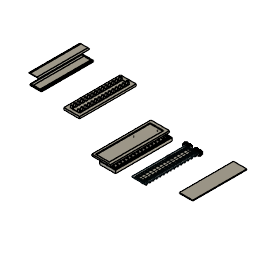
Prototype_caterpillar_body_mold_asser v11 (Autodesk Fusion 360 design; units mm, degrees)
Autodesk Fusion 360 part; units mm, degrees
note: some values were not read from the file. Chosen so that the rebuilt part matches the saved one: which bodies a step acts on; which face or edge a step refers to. Set by a fixed rule: which sketch regions a step uses.
(part 1 of 3)
sketch "Sketch1" plane through (0, 0, 0) normal (1, 0, 0) x (0, 1, 0)
  line L0 (0, 0) -> (0, 15)
  line L1 (0, 0) -> (5, 0)
  line L2 (5, 0) -> (13.6603, 15)
  line L3 (13.6603, 15) -> (16.3397, 15)
  line L4 (16.3397, 15) -> (25, 0)
  line L5 (25, 0) -> (30, 0)
  line L6 (30, 0) -> (38.6605, 15.0004)
  line L7 (0, 15) -> (38.6605, 15.0004)
  line L8 (12.7943, 13.5001) -> (17.2057, 13.5002)
  line L9 (12.7943, 13.5001) -> (12.7943, 15.0001)
  dimension "d1" = 15
  dimension "d4" = 5
  dimension "d5" = 120
  dimension "d9" = 15
  dimension "d11" = 120
  dimension "d12" = 20
  dimension "d13" = 5
  dimension "d14" = 2.6795
  dimension "d15" = 120
  dimension "d16" = 17.321
  dimension "d17" = 1.5
  constraint coincident L0.start L1.start
  constraint vertical L0
  constraint perpendicular L0 L1
  constraint perpendicular L0 L3
  constraint horizontal L5
  constraint coincident L2 L8.start
  constraint coincident L4 L8.end
  constraint parallel L7 L8
  constraint coincident L7 L9.end
  constraint perpendicular L7 L9
  measures "d1" distance of L0.start L0.end
  measures "d4" distance of L0.start L1.end
  measures "d5" angle of L1 L2
  measures "d9" distance of L1 L3
  measures "d11" angle of L4 L5
  measures "d12" distance of L1.end L4.end
  measures "d13" distance of L4.end L5.end
  measures "d14" distance of L2.end L3.end
  measures "d15" angle of L5 L6
  measures "d16" distance of L5.end L6.end
  measures "d17" distance of L7 L8
extrude "Extrude1" add sketch "Sketch1" along normal blind 60 contours L2 L7 L9 | L2 L3 L4 L7 L8 | L4 L5 L6 L7 makes body 1
sketch "Sketch2" plane through (0, 0, 0) normal (0, -1, 0) x (1, 0, 0)
  line L0 (0, 15) -> (0, 0)
  line L1 (0, 0) -> (60, 0)
  line L2 (60, 0) -> (60, 15)
  line L3 (60, 15) -> (0, 15)
  line L4 (0, 0) -> (15, 0)
  line L5 (60, 0) -> (45, 0)
  line L6 (15, 0) -> (30, 13.5)
  line L7 (45, 0) -> (30, 13.5)
  line L8 (15, 0) -> (45, 0)
  dimension "d23" = 15
  dimension "d24" = 15
  dimension "d28" = 138.013
  dimension "d29" = 138.013
  constraint coincident L0.end L1.start
  constraint coincident L1 L4.end
  constraint perpendicular L2 L4
  constraint coincident L1.end L2.start
  constraint coincident L1 L5.end
  constraint perpendicular L2 L5
  measures "d23" distance of L0.end L4.end
  measures "d24" distance of L1.end L5.end
  measures "d28" angle of L4 L6
  measures "d29" angle of L5 L7
extrude "Extrude2" cut sketch "Sketch2" along normal through all and the other way through all contours L1 L6 L7 L8 bodies 1
sketch "Sketch5" plane through (60, 0, 0) normal (1, 0, 0) x (0, 1, 0)
  line L0 (17.2057, 13.5002) -> (25, 0)
  line L1 (25, 0) -> (30, 0)
  line L2 (30, 0) -> (38.6605, 15.0004)
  line L3 (38.6605, 15.0004) -> (12.7943, 15.0001)
  line L4 (12.7943, 15.0001) -> (12.7943, 13.5001)
  line L5 (12.7943, 13.5001) -> (17.2057, 13.5002)
  line L6 (18.649, 15.0002) -> (24.7114, 4.4999)
  line L7 (24.7114, 4.4999) -> (30.2887, 4.5)
  line L8 (30.2887, 4.5) -> (36.3511, 15.0004)
  line L9 (18.649, 15.0002) -> (36.3511, 15.0004)
  dimension "d32" = 2
  dimension "d33" = 2
  dimension "d35" = 4.5
  constraint coincident L3 L6.start
  constraint parallel L3 L7
  constraint parallel L0 L6
  constraint parallel L2 L8
  constraint coincident L3 L8.end
  measures "d32" distance of L0 L6
  measures "d33" distance of L2 L8
  measures "d35" distance of L1.end L7
extrude "Extrude3" cut sketch "Sketch5" against normal blind 11 from surface at -4 contours L3 L6 L7 L8 L9 bodies 1
ref_plane "WorkPlane1" through (30, 25.7274, 7.5002) normal (1, 0, 0) x (0, 0, -1)
mirror "Mirror1" about plane through (30, 25.7274, 7.5002) normal (1, 0, 0) of "Extrude3"
pattern_linear "R-Pattern1" count 10 spacing 25 along (0, 1, 0) of bodies 1 makes body 2 at (35, 55.4504, 15.0003) makes body 3 at (35, 80.4504, 15.0003) makes body 4 at (35, 105.4504, 15.0003) makes body 5 at (35, 130.4504, 15.0003) makes body 6 at (35, 155.4504, 15.0003) makes body 7 at (35, 180.4504, 15.0003) makes body 8 at (35, 205.4504, 15.0003) makes body 9 at (35, 230.4504, 15.0003) makes body 10 at (35, 249.5497, 15.0003)
combine "Combine1" operation add target body 1 tool bodies 2 3 4 5 6 7 8 10 9
extrude "Extrude4" add sketch "Sketch1" along normal up to surface (60 mm away) contours L0 L1 L2 L7 L9 bodies 1
sketch "Sketch6" plane through (0, -0.0002, 15) normal (0, -0.000011, 1) x (1, 0, 0)
  line L0 (15, 18.6492) -> (4, 18.6492)
  line L1 (4, 18.6492) -> (4, 36.3512)
  line L2 (4, 36.3512) -> (15, 36.3512)
  line L3 (15, 36.3512) -> (15, 18.6492)
  line L4 (56, 18.6492) -> (45, 18.6492)
  line L5 (45, 18.6492) -> (45, 36.3512)
  line L6 (45, 36.3512) -> (56, 36.3512)
  line L7 (56, 36.3512) -> (56, 18.6492)
  line L8 (0, 38.6607) -> (0, 0.0002)
  line L9 (0, 0.0002) -> (60, 0.0002)
  line L10 (60, 0.0002) -> (60, 38.6607)
  line L11 (60, 38.6607) -> (0, 38.6607)
  line L12 (51.5, 36.3512) -> (49.5, 36.3512)
  line L13 (49.5, 36.3512) -> (49.5, 243.65)
  line L14 (49.5, 243.65) -> (51.5, 243.65)
  line L15 (51.5, 243.65) -> (51.5, 36.3512)
  line L16 (56, 243.65) -> (54.86, 243.65)
  line L17 (0, 263.5) -> (60, 263.5)
  line L18 (30, 263.5) -> (30, 202.2407)
  line L19 (8.5, 243.65) -> (8.5, 36.3512)
  line L20 (10.5, 36.3512) -> (10.5, 243.65)
  line L21 (8.5, 36.3512) -> (10.5, 36.3512)
  line L22 (10.5, 243.65) -> (8.5, 243.65)
  dimension "d48" = 2
  constraint vertical L13
  constraint horizontal L14
  constraint vertical L15
  constraint collinear L6 L12
  constraint horizontal L16
  constraint collinear L14 L16
  constraint midpoint L6 L12
  constraint horizontal L17
  constraint midpoint L17 L18.start
  constraint perpendicular L17 L18
  constraint symmetric L12.start L18 L19.end
  constraint symmetric L12.end L18 L20.start
  constraint symmetric L13.end L18 L20.end
  constraint symmetric L14.end L18 L19.start
  measures "d48" distance of L12.start L12.end
extrude "Extrude5" cut sketch "Sketch6" against normal blind 1 contours L2 L11 L19 L20 L21 | L11 L19 L20 L22 | L11 L13 L14 L15 | L6 L11 L12 L13 L15 bodies 1
extrude "Extrude6" add sketch "Sketch2" along normal blind 5 contours L0 L1 L2 L3 L4 L5 L6 L7 bodies 1
extrude "Extrude7" cut sketch "Sketch2" against normal blind 150 contours L1 L6 L7 L8 bodies 1
sketch "Sketch7" plane through (0, -0.0002, 15) normal (0, -0.000011, 1) x (1, 0, 0)
  line L0 (8.5, 36.3512) -> (8.5, 38.6607)
  line L1 (8.5, 38.6607) -> (0, 38.6607)
  line L2 (0, 38.6607) -> (0, 0.0002)
  line L3 (0, 0.0002) -> (60, 0.0002)
  line L4 (60, 0.0002) -> (60, 38.6607)
  line L5 (60, 38.6607) -> (51.5, 38.6607)
  line L6 (51.5, 38.6607) -> (51.5, 36.3512)
  line L7 (51.5, 36.3512) -> (56, 36.3512)
  line L8 (56, 36.3512) -> (56, 18.6492)
  line L9 (56, 18.6492) -> (45, 18.6492)
  line L10 (45, 18.6492) -> (45, 36.3512)
  line L11 (45, 36.3512) -> (49.5, 36.3512)
  line L12 (49.5, 36.3512) -> (49.5, 38.6607)
  line L13 (49.5, 38.6607) -> (10.5, 38.6607)
  line L14 (10.5, 38.6607) -> (10.5, 36.3512)
  line L15 (10.5, 36.3512) -> (15, 36.3512)
  line L16 (15, 36.3512) -> (15, 18.6492)
  line L17 (15, 18.6492) -> (4, 18.6492)
  line L18 (4, 18.6492) -> (4, 36.3512)
  line L19 (4, 36.3512) -> (8.5, 36.3512)
  line L20 (56, 18.6492) -> (45, 18.6492)
  line L21 (45, 18.6492) -> (45, 261.35)
  line L22 (45, 261.35) -> (56, 261.35)
  line L23 (56, 261.35) -> (56, 18.6492)
  line L24 (15, 18.6492) -> (4, 18.6492)
  line L25 (4, 18.6492) -> (4, 261.3513)
  line L26 (4, 261.3513) -> (15, 261.3513)
  line L27 (15, 261.3513) -> (15, 18.6492)
  line L28 (57, 262.35) -> (57, 17.6492)
  line L29 (57, 17.6492) -> (44, 17.6492)
  line L30 (44, 17.6492) -> (44, 262.35)
  line L31 (44, 262.35) -> (57, 262.35)
  line L32 (3, 262.3513) -> (16, 262.3513)
  line L33 (16, 262.3513) -> (16, 17.6492)
  line L34 (16, 17.6492) -> (3, 17.6492)
  line L35 (3, 17.6492) -> (3, 262.3513)
  dimension "d56" = -1
  dimension "d57" = -1
  constraint horizontal L20
  constraint vertical L21
  constraint horizontal L22
  constraint vertical L23
  constraint coincident L8.end L9.start
  constraint horizontal L24
  constraint vertical L25
  constraint horizontal L26
  constraint vertical L27
  constraint coincident L16.end L17.start
extrude "Extrude8" add sketch "Sketch7" along normal blind 2 contours L1 L13 L16 L17 L18 L24 L25 L27 L33 L34 L35 | L1 L13 L25 L26 L27 L32 L33 L35 | L5 L13 L21 L22 L23 L28 L30 L31 | L5 L8 L9 L10 L13 L20 L21 L23 L28 L29 L30 bodies 1
sketch "Sketch8" plane through (0, -0.0002, 14.9997) normal (0, -0.000011, 1) x (1, 0, 0)
  line L0 (8.5, 61.3512) -> (8.5, 63.6607)
  line L1 (8.5, 63.6607) -> (0, 63.6607)
  line L2 (0, 63.6607) -> (0, 38.6605)
  line L3 (0, 38.6605) -> (8.5, 38.6605)
  line L4 (8.5, 38.6605) -> (8.5, 43.6492)
  line L5 (8.5, 43.6492) -> (4, 43.6492)
  line L6 (4, 43.6492) -> (4, 61.3512)
  line L7 (4, 61.3512) -> (8.5, 61.3512)
  line L8 (8.5, 36.35) -> (4, 36.35)
  line L9 (4, 36.35) -> (4, 43.6492)
  line L10 (4, 43.6492) -> (8.5, 43.6492)
  line L11 (8.5, 43.6492) -> (8.5, 36.35)
  line L12 (4, 43.6492) -> (4, 36.35)
  line L13 (5, 42.6492) -> (7.5, 42.6492)
  line L14 (7.5, 42.6492) -> (7.5, 37.35)
  line L15 (7.5, 37.35) -> (5, 37.35)
  line L16 (5, 37.35) -> (5, 42.6492)
  line L17 (15, 19) -> (4, 19)
  line L18 (9.5, 19) -> (9.5, 28.6164)
  line L19 (11.5, 37.35) -> (14, 37.35)
  line L20 (14, 42.6492) -> (11.5, 42.6492)
  line L21 (14, 37.35) -> (14, 42.6492)
  line L22 (11.5, 42.6492) -> (11.5, 37.35)
  line L23 (60, 0) -> (0, 0)
  line L24 (30, 0) -> (30, 31)
  line L25 (0, 63.6605) -> (8.5, 63.6605)
  line L26 (8.5, 63.6605) -> (8.5, 68.6492)
  line L27 (11.5, 62.35) -> (14, 62.35)
  line L28 (8.5, 68.6492) -> (4, 68.6492)
  line L29 (5, 67.6492) -> (7.5, 67.6492)
  line L30 (7.5, 62.35) -> (5, 62.35)
  line L31 (5, 62.35) -> (5, 67.6492)
  line L32 (4, 68.6492) -> (8.5, 68.6492)
  line L33 (14, 67.6492) -> (11.5, 67.6492)
  line L34 (8.5, 61.35) -> (4, 61.35)
  line L35 (14, 62.35) -> (14, 67.6492)
  line L36 (8.5, 68.6492) -> (8.5, 61.35)
  line L37 (4, 68.6492) -> (4, 61.35)
  line L38 (11.5, 67.6492) -> (11.5, 62.35)
  line L39 (7.5, 67.6492) -> (7.5, 62.35)
  line L40 (4, 61.35) -> (4, 68.6492)
  line L41 (0, 88.6605) -> (8.5, 88.6605)
  line L42 (8.5, 88.6605) -> (8.5, 93.6492)
  line L43 (11.5, 87.35) -> (14, 87.35)
  line L44 (8.5, 93.6492) -> (4, 93.6492)
  line L45 (5, 92.6492) -> (7.5, 92.6492)
  line L46 (7.5, 87.35) -> (5, 87.35)
  line L47 (5, 87.35) -> (5, 92.6492)
  line L48 (4, 93.6492) -> (8.5, 93.6492)
  line L49 (14, 92.6492) -> (11.5, 92.6492)
  line L50 (8.5, 86.35) -> (4, 86.35)
  line L51 (14, 87.35) -> (14, 92.6492)
  line L52 (8.5, 93.6492) -> (8.5, 86.35)
  line L53 (4, 93.6492) -> (4, 86.35)
  line L54 (11.5, 92.6492) -> (11.5, 87.35)
  line L55 (7.5, 92.6492) -> (7.5, 87.35)
  line L56 (4, 86.35) -> (4, 93.6492)
  line L57 (0, 113.6605) -> (8.5, 113.6605)
  line L58 (8.5, 113.6605) -> (8.5, 118.6492)
  line L59 (11.5, 112.35) -> (14, 112.35)
  line L60 (8.5, 118.6492) -> (4, 118.6492)
  line L61 (5, 117.6492) -> (7.5, 117.6492)
  line L62 (7.5, 112.35) -> (5, 112.35)
  line L63 (5, 112.35) -> (5, 117.6492)
  line L64 (4, 118.6492) -> (8.5, 118.6492)
  line L65 (14, 117.6492) -> (11.5, 117.6492)
  line L66 (8.5, 111.35) -> (4, 111.35)
  line L67 (14, 112.35) -> (14, 117.6492)
  line L68 (8.5, 118.6492) -> (8.5, 111.35)
  line L69 (4, 118.6492) -> (4, 111.35)
  line L70 (11.5, 117.6492) -> (11.5, 112.35)
  line L71 (7.5, 117.6492) -> (7.5, 112.35)
  line L72 (4, 111.35) -> (4, 118.6492)
  line L73 (0, 138.6605) -> (8.5, 138.6605)
  line L74 (8.5, 138.6605) -> (8.5, 143.6492)
  line L75 (11.5, 137.35) -> (14, 137.35)
  line L76 (8.5, 143.6492) -> (4, 143.6492)
  line L77 (5, 142.6492) -> (7.5, 142.6492)
  line L78 (7.5, 137.35) -> (5, 137.35)
  line L79 (5, 137.35) -> (5, 142.6492)
  line L80 (4, 143.6492) -> (8.5, 143.6492)
  line L81 (14, 142.6492) -> (11.5, 142.6492)
  line L82 (8.5, 136.35) -> (4, 136.35)
  line L83 (14, 137.35) -> (14, 142.6492)
  line L84 (8.5, 143.6492) -> (8.5, 136.35)
  line L85 (4, 143.6492) -> (4, 136.35)
  line L86 (11.5, 142.6492) -> (11.5, 137.35)
  line L87 (7.5, 142.6492) -> (7.5, 137.35)
  line L88 (4, 136.35) -> (4, 143.6492)
  line L89 (0, 163.6605) -> (8.5, 163.6605)
  line L90 (8.5, 163.6605) -> (8.5, 168.6492)
  line L91 (11.5, 162.35) -> (14, 162.35)
  line L92 (8.5, 168.6492) -> (4, 168.6492)
  line L93 (5, 167.6492) -> (7.5, 167.6492)
  line L94 (7.5, 162.35) -> (5, 162.35)
  line L95 (5, 162.35) -> (5, 167.6492)
  line L96 (4, 168.6492) -> (8.5, 168.6492)
  line L97 (14, 167.6492) -> (11.5, 167.6492)
  line L98 (8.5, 161.35) -> (4, 161.35)
  line L99 (14, 162.35) -> (14, 167.6492)
  line L100 (8.5, 168.6492) -> (8.5, 161.35)
  line L101 (4, 168.6492) -> (4, 161.35)
  line L102 (11.5, 167.6492) -> (11.5, 162.35)
  line L103 (7.5, 167.6492) -> (7.5, 162.35)
  line L104 (4, 161.35) -> (4, 168.6492)
  line L105 (0, 188.6605) -> (8.5, 188.6605)
  line L106 (8.5, 188.6605) -> (8.5, 193.6492)
  line L107 (11.5, 187.35) -> (14, 187.35)
  line L108 (8.5, 193.6492) -> (4, 193.6492)
  line L109 (5, 192.6492) -> (7.5, 192.6492)
  line L110 (7.5, 187.35) -> (5, 187.35)
  line L111 (5, 187.35) -> (5, 192.6492)
  line L112 (4, 193.6492) -> (8.5, 193.6492)
  line L113 (14, 192.6492) -> (11.5, 192.6492)
  line L114 (8.5, 186.35) -> (4, 186.35)
  line L115 (14, 187.35) -> (14, 192.6492)
  line L116 (8.5, 193.6492) -> (8.5, 186.35)
  line L117 (4, 193.6492) -> (4, 186.35)
  line L118 (11.5, 192.6492) -> (11.5, 187.35)
  line L119 (7.5, 192.6492) -> (7.5, 187.35)
  line L120 (4, 186.35) -> (4, 193.6492)
  line L121 (0, 213.6605) -> (8.5, 213.6605)
  line L122 (8.5, 213.6605) -> (8.5, 218.6492)
  line L123 (11.5, 212.35) -> (14, 212.35)
  line L124 (8.5, 218.6492) -> (4, 218.6492)
  line L125 (5, 217.6492) -> (7.5, 217.6492)
  line L126 (7.5, 212.35) -> (5, 212.35)
  line L127 (5, 212.35) -> (5, 217.6492)
  line L128 (4, 218.6492) -> (8.5, 218.6492)
  line L129 (14, 217.6492) -> (11.5, 217.6492)
  line L130 (8.5, 211.35) -> (4, 211.35)
  line L131 (14, 212.35) -> (14, 217.6492)
  line L132 (8.5, 218.6492) -> (8.5, 211.35)
  line L133 (4, 218.6492) -> (4, 211.35)
  line L134 (11.5, 217.6492) -> (11.5, 212.35)
  line L135 (7.5, 217.6492) -> (7.5, 212.35)
  line L136 (4, 211.35) -> (4, 218.6492)
  line L137 (0, 238.6605) -> (8.5, 238.6605)
  line L138 (8.5, 238.6605) -> (8.5, 243.6492)
  line L139 (11.5, 237.35) -> (14, 237.35)
  line L140 (8.5, 243.6492) -> (4, 243.6492)
  line L141 (5, 242.6492) -> (7.5, 242.6492)
  line L142 (7.5, 237.35) -> (5, 237.35)
  line L143 (5, 237.35) -> (5, 242.6492)
  line L144 (4, 243.6492) -> (8.5, 243.6492)
  line L145 (14, 242.6492) -> (11.5, 242.6492)
  line L146 (8.5, 236.35) -> (4, 236.35)
  line L147 (14, 237.35) -> (14, 242.6492)
  line L148 (8.5, 243.6492) -> (8.5, 236.35)
  line L149 (4, 243.6492) -> (4, 236.35)
  line L150 (11.5, 242.6492) -> (11.5, 237.35)
  line L151 (7.5, 242.6492) -> (7.5, 237.35)
  line L152 (4, 236.35) -> (4, 243.6492)
  line L153 (45, 19) -> (56, 19)
  line L154 (48.5, 37.35) -> (46, 37.35)
  line L155 (56, 93.6492) -> (56, 86.35)
  line L156 (52.5, 187.35) -> (55, 187.35)
  line L157 (56, 118.6492) -> (56, 111.35)
  line L158 (46, 187.35) -> (46, 192.6492)
  line L159 (51.5, 136.35) -> (56, 136.35)
  line L160 (52.5, 37.35) -> (55, 37.35)
  line L161 (52.5, 167.6492) -> (52.5, 162.35)
  line L162 (56, 43.6492) -> (56, 36.35)
  line L163 (51.5, 118.6492) -> (51.5, 111.35)
  line L164 (55, 37.35) -> (55, 42.6492)
  line L165 (51.5, 61.3512) -> (51.5, 63.6607)
  line L166 (60, 113.6605) -> (51.5, 113.6605)
  line L167 (51.5, 88.6605) -> (51.5, 93.6492)
  line L168 (56, 61.3512) -> (51.5, 61.3512)
  line L169 (52.5, 42.6492) -> (52.5, 37.35)
  line L170 (48.5, 142.6492) -> (48.5, 137.35)
  line L171 (55, 237.35) -> (55, 242.6492)
  line L172 (51.5, 43.6492) -> (51.5, 36.35)
  line L173 (51.5, 63.6607) -> (60, 63.6607)
  line L174 (46, 42.6492) -> (48.5, 42.6492)
  line L175 (60, 163.6605) -> (51.5, 163.6605)
  line L176 (51.5, 86.35) -> (56, 86.35)
  line L177 (56, 143.6492) -> (56, 136.35)
  line L178 (50.5, 19) -> (50.5, 28.6164)
  line L179 (55, 167.6492) -> (52.5, 167.6492)
  line L180 (60, 38.6605) -> (51.5, 38.6605)
  line L181 (51.5, 188.6605) -> (51.5, 193.6492)
  line L182 (51.5, 36.35) -> (56, 36.35)
  line L183 (56, 168.6492) -> (56, 161.35)
  line L184 (48.5, 87.35) -> (46, 87.35)
  line L185 (46, 112.35) -> (46, 117.6492)
  line L186 (51.5, 138.6605) -> (51.5, 143.6492)
  line L187 (56, 36.35) -> (56, 43.6492)
  line L188 (55, 42.6492) -> (52.5, 42.6492)
  line L189 (46, 167.6492) -> (48.5, 167.6492)
  line L190 (51.5, 38.6605) -> (51.5, 43.6492)
  line L191 (51.5, 111.35) -> (56, 111.35)
  line L192 (56, 143.6492) -> (51.5, 143.6492)
  line L193 (48.5, 112.35) -> (46, 112.35)
  line L194 (46, 37.35) -> (46, 42.6492)
  line L195 (51.5, 43.6492) -> (56, 43.6492)
  line L196 (56, 43.6492) -> (51.5, 43.6492)
  line L197 (52.5, 112.35) -> (55, 112.35)
  line L198 (48.5, 137.35) -> (46, 137.35)
  line L199 (60, 188.6605) -> (51.5, 188.6605)
  line L200 (60, 138.6605) -> (51.5, 138.6605)
  line L201 (60, 63.6607) -> (60, 38.6605)
  line L202 (56, 43.6492) -> (56, 61.3512)
  line L203 (48.5, 42.6492) -> (48.5, 37.35)
  line L204 (56, 168.6492) -> (51.5, 168.6492)
  line L205 (55, 187.35) -> (55, 192.6492)
  line L206 (55, 192.6492) -> (52.5, 192.6492)
  line L207 (56, 86.35) -> (56, 93.6492)
  line L208 (52.5, 237.35) -> (55, 237.35)
  line L209 (46, 237.35) -> (46, 242.6492)
  line L210 (48.5, 162.35) -> (46, 162.35)
  line L211 (56, 193.6492) -> (51.5, 193.6492)
  line L212 (48.5, 242.6492) -> (48.5, 237.35)
  line L213 (52.5, 137.35) -> (55, 137.35)
  line L214 (55, 112.35) -> (55, 117.6492)
  line L215 (51.5, 193.6492) -> (56, 193.6492)
  line L216 (52.5, 142.6492) -> (52.5, 137.35)
  line L217 (51.5, 218.6492) -> (51.5, 211.35)
  line L218 (46, 192.6492) -> (48.5, 192.6492)
  line L219 (55, 142.6492) -> (52.5, 142.6492)
  line L220 (52.5, 117.6492) -> (52.5, 112.35)
  line L221 (56, 243.6492) -> (51.5, 243.6492)
  line L222 (48.5, 117.6492) -> (48.5, 112.35)
  line L223 (51.5, 163.6605) -> (51.5, 168.6492)
  line L224 (56, 243.6492) -> (56, 236.35)
  line L225 (48.5, 217.6492) -> (48.5, 212.35)
  line L226 (46, 242.6492) -> (48.5, 242.6492)
  line L227 (55, 87.35) -> (55, 92.6492)
  line L228 (46, 162.35) -> (46, 167.6492)
  line L229 (52.5, 212.35) -> (55, 212.35)
  line L230 (51.5, 68.6492) -> (56, 68.6492)
  line L231 (60, 63.6605) -> (51.5, 63.6605)
  line L232 (52.5, 242.6492) -> (52.5, 237.35)
  line L233 (46, 117.6492) -> (48.5, 117.6492)
  line L234 (52.5, 162.35) -> (55, 162.35)
  line L235 (55, 137.35) -> (55, 142.6492)
  line L236 (55, 117.6492) -> (52.5, 117.6492)
  line L237 (46, 212.35) -> (46, 217.6492)
  line L238 (51.5, 213.6605) -> (51.5, 218.6492)
  line L239 (51.5, 186.35) -> (56, 186.35)
  line L240 (52.5, 92.6492) -> (52.5, 87.35)
  line L241 (48.5, 192.6492) -> (48.5, 187.35)
  line L242 (46, 87.35) -> (46, 92.6492)
  line L243 (51.5, 238.6605) -> (51.5, 243.6492)
  line L244 (46, 142.6492) -> (48.5, 142.6492)
  line L245 (51.5, 143.6492) -> (56, 143.6492)
  line L246 (56, 186.35) -> (56, 193.6492)
  line L247 (56, 161.35) -> (56, 168.6492)
  line L248 (56, 193.6492) -> (56, 186.35)
  line L249 (56, 111.35) -> (56, 118.6492)
  line L250 (51.5, 168.6492) -> (56, 168.6492)
  line L251 (52.5, 192.6492) -> (52.5, 187.35)
  line L252 (55, 162.35) -> (55, 167.6492)
  line L253 (48.5, 187.35) -> (46, 187.35)
  line L254 (56, 118.6492) -> (51.5, 118.6492)
  line L255 (55, 212.35) -> (55, 217.6492)
  line L256 (56, 136.35) -> (56, 143.6492)
  line L257 (55, 217.6492) -> (52.5, 217.6492)
  line L258 (51.5, 193.6492) -> (51.5, 186.35)
  line L259 (56, 218.6492) -> (56, 211.35)
  line L260 (52.5, 67.6492) -> (52.5, 62.35)
  line L261 (51.5, 243.6492) -> (56, 243.6492)
  line L262 (51.5, 143.6492) -> (51.5, 136.35)
  line L263 (51.5, 236.35) -> (56, 236.35)
  line L264 (46, 67.6492) -> (48.5, 67.6492)
  line L265 (56, 68.6492) -> (56, 61.35)
  line L266 (48.5, 167.6492) -> (48.5, 162.35)
  line L267 (55, 92.6492) -> (52.5, 92.6492)
  line L268 (51.5, 168.6492) -> (51.5, 161.35)
  line L269 (46, 137.35) -> (46, 142.6492)
  line L270 (56, 68.6492) -> (51.5, 68.6492)
  line L271 (52.5, 62.35) -> (55, 62.35)
  line L272 (51.5, 161.35) -> (56, 161.35)
  line L273 (48.5, 237.35) -> (46, 237.35)
  line L274 (51.5, 113.6605) -> (51.5, 118.6492)
  line L275 (51.5, 118.6492) -> (56, 118.6492)
  line L276 (51.5, 61.35) -> (56, 61.35)
  line L277 (51.5, 93.6492) -> (51.5, 86.35)
  line L278 (52.5, 87.35) -> (55, 87.35)
  line L279 (60, 238.6605) -> (51.5, 238.6605)
  line L280 (51.5, 243.6492) -> (51.5, 236.35)
  line L281 (51.5, 68.6492) -> (51.5, 61.35)
  line L282 (56, 93.6492) -> (51.5, 93.6492)
  line L283 (51.5, 93.6492) -> (56, 93.6492)
  line L284 (51.5, 218.6492) -> (56, 218.6492)
  line L285 (46, 62.35) -> (46, 67.6492)
  line L286 (56, 61.35) -> (56, 68.6492)
  line L287 (48.5, 62.35) -> (46, 62.35)
  line L288 (60, 213.6605) -> (51.5, 213.6605)
  line L289 (55, 242.6492) -> (52.5, 242.6492)
  line L290 (51.5, 63.6605) -> (51.5, 68.6492)
  line L291 (56, 218.6492) -> (51.5, 218.6492)
  line L292 (48.5, 212.35) -> (46, 212.35)
  line L293 (46, 217.6492) -> (48.5, 217.6492)
  line L294 (48.5, 92.6492) -> (48.5, 87.35)
  line L295 (55, 67.6492) -> (52.5, 67.6492)
  line L296 (51.5, 211.35) -> (56, 211.35)
  line L297 (46, 92.6492) -> (48.5, 92.6492)
  line L298 (52.5, 217.6492) -> (52.5, 212.35)
  line L299 (56, 236.35) -> (56, 243.6492)
  line L300 (60, 88.6605) -> (51.5, 88.6605)
  line L301 (48.5, 67.6492) -> (48.5, 62.35)
  line L302 (55, 62.35) -> (55, 67.6492)
  line L303 (56, 211.35) -> (56, 218.6492)
  dimension "d60" = 4.5
  dimension "d61" = 7.2992
  dimension "d64" = 1
  dimension "d67" = 0
  dimension "d68" = 25
  constraint horizontal L8
  constraint vertical L9
  constraint horizontal L10
  constraint vertical L11
  constraint coincident L5.end L6.start
  constraint horizontal L17
  constraint midpoint L17 L18.start
  constraint perpendicular L17 L18
  constraint symmetric L13.start L18 L20.start
  constraint symmetric L13.end L18 L20.end
  constraint symmetric L14.end L18 L19.start
  constraint symmetric L15.end L18 L19.end
  constraint coincident L23.end origin
  constraint horizontal L23
  constraint midpoint L23 L24.start
  constraint perpendicular L23 L24
  constraint symmetric L0.start L24 L165.start
  constraint symmetric L0.end L24 L165.end
  constraint symmetric L1.end L24 L173.end
  constraint symmetric L2.end L24 L180.start
  constraint symmetric L3.end L24 L180.end
  constraint symmetric L4.end L24 L172.start
  constraint symmetric L5.end L24 L162.start
  constraint symmetric L6.end L24 L168.start
  constraint symmetric L8.start L24 L172.end
  constraint symmetric L8.end L24 L162.end
  constraint symmetric L13.start L24 L164.end
  constraint symmetric L13.end L24 L169.start
  constraint symmetric L14.end L24 L160.start
  constraint symmetric L15.end L24 L160.end
  constraint symmetric L17.start L24 L153.start
  constraint symmetric L17.end L24 L153.end
  constraint symmetric L18.start L24 L178.start
  constraint symmetric L18.end L24 L178.end
  constraint symmetric L20.start L24 L174.start
  constraint symmetric L19.start L24 L154.start
  constraint symmetric L19.end L24 L154.end
  constraint symmetric L20.end L24 L174.end
  constraint symmetric L24 L25.start L231.start
  constraint symmetric L24 L25.end L231.end
  constraint symmetric L24 L28.end L230.end
  constraint symmetric L24 L26.end L230.start
  constraint symmetric L24 L30.start L260.end
  constraint symmetric L24 L27.start L287.start
  constraint symmetric L24 L27.end L285.start
  constraint symmetric L24 L29.start L295.start
  constraint symmetric L24 L29.end L260.start
  constraint symmetric L24 L30.end L271.end
  constraint symmetric L24 L34.end L265.end
  constraint symmetric L24 L33.end L264.end
  constraint symmetric L24 L33.start L264.start
  constraint symmetric L24 L34.start L276.start
  constraint symmetric L24 L41.start L300.start
  constraint symmetric L24 L41.end L167.start
  constraint symmetric L24 L44.end L155.start
  constraint symmetric L24 L42.end L167.end
  constraint symmetric L24 L46.start L240.end
  constraint symmetric L24 L43.start L184.start
  constraint symmetric L24 L43.end L184.end
  constraint symmetric L24 L45.start L227.end
  constraint symmetric L24 L45.end L240.start
  constraint symmetric L24 L46.end L227.start
  constraint symmetric L24 L50.end L155.end
  constraint symmetric L24 L49.end L294.start
  constraint symmetric L24 L49.start L242.end
  constraint symmetric L24 L50.start L176.start
  constraint symmetric L24 L57.start L166.start
  constraint symmetric L24 L57.end L166.end
  constraint symmetric L24 L60.end L157.start
  constraint symmetric L24 L58.end L163.start
  constraint symmetric L24 L62.start L197.start
  constraint symmetric L24 L59.start L193.start
  constraint symmetric L24 L59.end L185.start
  constraint symmetric L24 L61.start L214.end
  constraint symmetric L24 L61.end L220.start
  constraint symmetric L24 L62.end L197.end
  constraint symmetric L24 L66.end L157.end
  constraint symmetric L24 L65.end L222.start
  constraint symmetric L24 L65.start L185.end
  constraint symmetric L24 L66.start L163.end
  constraint symmetric L24 L73.start L200.start
  constraint symmetric L24 L73.end L186.start
  constraint symmetric L24 L76.end L177.start
  constraint symmetric L24 L74.end L186.end
  constraint symmetric L24 L78.start L213.start
  constraint symmetric L24 L75.start L170.end
  constraint symmetric L24 L75.end L198.end
  constraint symmetric L24 L77.start L219.start
  constraint symmetric L24 L77.end L216.start
  constraint symmetric L24 L78.end L213.end
  constraint symmetric L24 L82.end L159.end
  constraint symmetric L24 L81.end L170.start
  constraint symmetric L24 L81.start L244.start
  constraint symmetric L24 L82.start L159.start
  constraint symmetric L24 L89.start L175.start
  constraint symmetric L24 L89.end L175.end
  constraint symmetric L24 L92.end L183.start
  constraint symmetric L24 L90.end L204.end
  constraint symmetric L24 L94.start L161.end
  constraint symmetric L24 L91.start L210.start
  constraint symmetric L24 L91.end L210.end
  constraint symmetric L24 L93.start L179.start
  constraint symmetric L24 L93.end L161.start
  constraint symmetric L24 L94.end L234.end
  constraint symmetric L24 L98.end L183.end
  constraint symmetric L24 L97.end L189.end
  constraint symmetric L24 L97.start L189.start
  constraint symmetric L24 L98.start L268.end
  constraint symmetric L24 L105.start L199.start
  constraint symmetric L24 L105.end L181.start
  constraint symmetric L24 L108.end L211.start
  constraint symmetric L24 L106.end L181.end
  constraint symmetric L24 L110.start L156.start
  constraint symmetric L24 L107.start L241.end
  constraint symmetric L24 L107.end L158.start
  constraint symmetric L24 L109.start L205.end
  constraint symmetric L24 L109.end L206.end
  constraint symmetric L24 L110.end L156.end
  constraint symmetric L24 L114.end L239.end
  constraint symmetric L24 L113.end L218.end
  constraint symmetric L24 L113.start L158.end
  constraint symmetric L24 L114.start L239.start
  constraint symmetric L24 L121.start L288.start
  constraint symmetric L24 L121.end L238.start
  constraint symmetric L24 L124.end L259.start
  constraint symmetric L24 L122.end L217.start
  constraint symmetric L24 L126.start L229.start
  constraint symmetric L24 L123.start L225.end
  constraint symmetric L24 L123.end L237.start
  constraint symmetric L24 L125.start L255.end
  constraint symmetric L24 L125.end L257.end
  constraint symmetric L24 L126.end L229.end
  constraint symmetric L24 L130.end L259.end
  constraint symmetric L24 L129.end L225.start
  constraint symmetric L24 L129.start L237.end
  constraint symmetric L24 L130.start L217.end
  constraint symmetric L24 L137.start L279.start
  constraint symmetric L24 L137.end L243.start
  constraint symmetric L24 L140.end L221.start
  constraint symmetric L24 L138.end L221.end
  constraint symmetric L24 L142.start L208.start
  constraint symmetric L24 L139.start L212.end
  constraint symmetric L24 L139.end L209.start
  constraint symmetric L24 L141.start L171.end
  constraint symmetric L24 L141.end L232.start
  constraint symmetric L24 L142.end L171.start
  constraint symmetric L24 L146.end L224.end
  constraint symmetric L24 L145.end L212.start
  constraint symmetric L24 L145.start L209.end
  constraint symmetric L24 L146.start L263.start
  measures "d60" distance of L8.start L8.end
  measures "d61" distance of L8.start L4.end
extrude "Extrude9" add sketch "Sketch8" along normal blind 2 contours L1 L25 L30 L31 L39 | L1 L25 L29 L31 L39 | L3 L13 L14 L16 | L3 L14 L15 L16 | L19 L20 L21 L22 | L27 L33 L35 L38 | L41 L45 L47 L55 | L41 L46 L47 L55 | L43 L49 L51 L54 | L57 L61 L63 L71 | L57 L62 L63 L71 | L59 L65 L67 L70 | L73 L77 L79 L87 | L73 L78 L79 L87 | L75 L81 L83 L86 | L89 L93 L95 L103 | L89 L94 L95 L103 | L91 L97 L99 L102 | L105 L109 L111 L119 | L105 L110 L111 L119 | L107 L113 L115 L118 | L121 L125 L127 L135 | L121 L126 L127 L135 | L123 L129 L131 L134 | L137 L141 L143 L151 | L137 L142 L143 L151 | L139 L145 L147 L150 | L154 L174 L194 L203 | L227 L240 L267 L300 | L227 L240 L278 L300 | L156 L199 L205 L251 | L199 L205 L206 L251 | L166 L197 L214 L220 | L166 L214 L220 L236 | L158 L218 L241 L253 | L200 L216 L219 L235 | L200 L213 L216 L235 | L160 L164 L169 L180 | L164 L169 L180 L188 | L173 L231 L260 L271 L302 | L173 L231 L260 L295 L302 | L161 L175 L179 L252 | L161 L175 L234 L252 | L170 L198 L244 L269 | L171 L208 L232 L279 | L171 L232 L279 L289 | L184 L242 L294 L297 | L185 L193 L222 L233 | L189 L210 L228 L266 | L209 L212 L226 L273 | L255 L257 L288 L298 | L229 L255 L288 L298 | L225 L237 L292 L293 | L264 L285 L287 L301 bodies 1 makes body 11 at (46.8333, 239.1162, 15.0024) makes body 12 at (53.3333, 215.8826, 15.0021) makes body 13 at (53.3333, 189.1162, 17.0018) makes body 14 at (46.8333, 165.8826, 17.0016) makes body 15 at (46.8333, 140.8826, 17.0013) makes body 16 at (5.8333, 90.8826, 17.0007) makes body 17 at (12.3333, 90.8826, 17.0007) makes body 18 at (12.3333, 115.8826, 17.001) makes body 19 at (53.3333, 115.8826, 17.001) makes body 20 at (12.3333, 140.8826, 17.0013) makes body 21 at (12.3333, 165.8826, 17.0016) makes body 22 at (12.3333, 190.8826, 17.0018) makes body 23 at (46.8333, 215.8826, 15.0021) makes body 24 at (53.3333, 240.8826, 15.0024) makes body 25 at (12.3333, 240.8826, 15.0024) makes body 26 at (5.8333, 215.8826, 15.0021) makes body 27 at (46.8333, 189.1162, 17.0018) makes body 28 at (53.3333, 165.8826, 17.0016) makes body 29 at (53.3333, 140.8826, 17.0013) makes body 30 at (53.3333, 90.8826, 17.0007) makes body 31 at (46.8333, 89.1162, 17.0007) makes body 32 at (46.8333, 114.1162, 17.001) makes body 33 at (5.8333, 115.8826, 17.001) makes body 34 at (5.8333, 140.8826, 17.0013) makes body 35 at (5.8333, 165.8826, 17.0016) makes body 36 at (5.8333, 189.1162, 17.0018) makes body 37 at (12.3333, 215.8826, 15.0021) makes body 38 at (5.8333, 240.8826, 15.0024)
sketch "Sketch9" plane through (0, 0, 0) normal (0, 0, 1) x (1, 0, 0)
  line L0 (60, 263.6606) -> (0, 263.6606)
  line L1 (0, 263.6606) -> (0, -5)
  line L2 (0, -5) -> (60, -5)
  line L3 (60, -5) -> (60, 263.6606)
  line L4 (-5, -10) -> (65, -10)
  line L5 (65, -10) -> (65, 268.6606)
  line L6 (65, 268.6606) -> (-5, 268.6606)
  line L7 (-5, 268.6606) -> (-5, -10)
  dimension "d71" = 5
  constraint horizontal L0
  constraint vertical L1
  constraint horizontal L2
  constraint vertical L3
ref_plane "WorkPlane2" through (250, 0, 0) normal (1, 0, 0) x (0, 1, 0)
sketch "Sketch10" plane through (250, 0, 0) normal (1, 0, 0) x (0, 1, 0)
  line L0 (0, 0) -> (0, 15)
  line L1 (0, 15) -> (250, 15)
  line L2 (0, 0) -> (10, 0)
  line L3 (10, 0) -> (14.7316, 13)
  line L4 (14.7316, 13) -> (17.2684, 13)
  line L5 (17.2684, 13) -> (22, 0)
  line L6 (22, 0) -> (27, 0)
  line L7 (27, 0) -> (31.7316, 13)
  line L8 (31.7316, 13) -> (34.2684, 13)
  line L9 (34.2684, 13) -> (39, 0)
  line L10 (39, 0) -> (44, 0)
  line L11 (44, 0) -> (48.7316, 13)
  line L12 (48.7316, 13) -> (51.2684, 13)
  line L13 (51.2684, 13) -> (56, 0)
  line L14 (56, 0) -> (61, 0)
  line L15 (61, 0) -> (65.7316, 13)
  line L16 (65.7316, 13) -> (68.2684, 13)
  line L17 (68.2684, 13) -> (73, 0)
  line L18 (73, 0) -> (78, 0)
  line L19 (78, 0) -> (82.7316, 13)
  line L20 (82.7316, 13) -> (85.2684, 13)
  line L21 (85.2684, 13) -> (90, 0)
  line L22 (90, 0) -> (95, 0)
  line L23 (95, 0) -> (99.7316, 13)
  line L24 (99.7316, 13) -> (102.2684, 13)
  line L25 (102.2684, 13) -> (107, 0)
  line L26 (107, 0) -> (112, 0)
  line L27 (112, 0) -> (116.7316, 13)
  line L28 (116.7316, 13) -> (119.2684, 13)
  line L29 (119.2684, 13) -> (124, 0)
  line L30 (124, 0) -> (129, 0)
  line L31 (129, 0) -> (133.7316, 13)
  line L32 (133.7316, 13) -> (136.2684, 13)
  line L33 (136.2684, 13) -> (141, 0)
  line L34 (141, 0) -> (146, 0)
  line L35 (146, 0) -> (150.7316, 13)
  line L36 (150.7316, 13) -> (153.2684, 13)
  line L37 (153.2684, 13) -> (158, 0)
  line L38 (158, 0) -> (163, 0)
  line L39 (163, 0) -> (167.7316, 13)
  line L40 (167.7316, 13) -> (170.2684, 13)
  line L41 (170.2684, 13) -> (175, 0)
  line L42 (175, 0) -> (180, 0)
  line L43 (180, 0) -> (184.7316, 13)
  line L44 (184.7316, 13) -> (187.2684, 13)
  line L45 (187.2684, 13) -> (192, 0)
  line L46 (192, 0) -> (197, 0)
  line L47 (197, 0) -> (201.7316, 13)
  line L48 (201.7316, 13) -> (204.2684, 13)
  line L49 (204.2684, 13) -> (209, 0)
  line L50 (209, 0) -> (214, 0)
  line L51 (214, 0) -> (218.7316, 13)
  line L52 (218.7316, 13) -> (221.2684, 13)
  line L53 (221.2684, 13) -> (226, 0)
  line L54 (226, 0) -> (231, 0)
  line L55 (231, 0) -> (235.7316, 13)
  line L56 (235.7316, 13) -> (238.2684, 13)
  line L57 (238.2684, 13) -> (243, 0)
  line L58 (243, 0) -> (248, 0)
  line L59 (250, 15) -> (250, 0)
  line L60 (250, 0) -> (248, 0)
  dimension "d75" = 250
  dimension "d76" = 15
  dimension "d77" = 2
  dimension "d78" = 110
  dimension "d79" = 110
  dimension "d80" = 12
  dimension "d81" = 5
  dimension "d82" = 10
  dimension "d85" = 17
  dimension "d86" = 0
  constraint coincident L0.start L2.start
  constraint vertical L0
  constraint perpendicular L0 L1
  constraint perpendicular L0 L2
  constraint perpendicular L0 L4
  constraint horizontal L6
  constraint collinear L2 L6
  constraint perpendicular L1 L59
  constraint perpendicular L59 L60
  measures "d75" distance of L0.end L1.end
  measures "d76" distance of L0.start L0.end
  measures "d77" distance of L1 L4
  measures "d78" angle of L2 L3
  measures "d79" angle of L5 L6
  measures "d80" distance of L2.end L5.end
  measures "d81" distance of L5.end L6.end
  measures "d82" distance of L0.start L2.end
extrude "Extrude11" add sketch "Sketch10" along normal blind 50 separate body makes body 39
sketch "Sketch11" plane through (0, 0, 0) normal (0, -1, 0) x (1, 0, 0)
  line L0 (250, 15) -> (250, 0)
  line L1 (250, 0) -> (300, 0)
  line L2 (300, 0) -> (300, 15)
  line L3 (300, 15) -> (250, 15)
  line L4 (250, 0) -> (263, 0)
  line L5 (300, 0) -> (287, 0)
  line L6 (275, 0) -> (275, 13)
  line L7 (263, 0) -> (275, 13)
  line L8 (287, 0) -> (275, 13)
  dimension "d89" = 13
  dimension "d90" = 13
  dimension "d91" = 13
  constraint coincident L0.end L1.start
  constraint coincident L1 L4.end
  constraint coincident L1.end L2.start
  constraint coincident L1 L5.end
  constraint midpoint L1 L6.start
  constraint perpendicular L1 L6
  measures "d89" distance of L0.end L4.end
  measures "d90" distance of L1.end L5.end
  measures "d91" distance of L6.start L6.end
extrude "Extrude12" cut sketch "Sketch11" along normal through all and the other way through all contours L1 L6 L7 | L1 L6 L8 bodies 39
sketch "Sketch12" plane through (300, 0, 0) normal (1, 0, 0) x (0, 1, 0)
  line L0 (0, 0) -> (10, 0)
  line L1 (10, 0) -> (14.7316, 13)
  line L2 (14.7316, 13) -> (17.2684, 13)
  line L3 (17.2684, 13) -> (22, 0)
  line L4 (22, 0) -> (27, 0)
  line L5 (27, 0) -> (31.7316, 13)
  line L6 (31.7316, 13) -> (34.2684, 13)
  line L7 (34.2684, 13) -> (39, 0)
  line L8 (39, 0) -> (44, 0)
  line L9 (44, 0) -> (48.7316, 13)
  line L10 (48.7316, 13) -> (51.2684, 13)
  line L11 (51.2684, 13) -> (56, 0)
  line L12 (56, 0) -> (61, 0)
  line L13 (61, 0) -> (65.7316, 13)
  line L14 (65.7316, 13) -> (68.2684, 13)
  line L15 (68.2684, 13) -> (73, 0)
  line L16 (73, 0) -> (78, 0)
  line L17 (78, 0) -> (82.7316, 13)
  line L18 (82.7316, 13) -> (85.2684, 13)
  line L19 (85.2684, 13) -> (90, 0)
  line L20 (90, 0) -> (95, 0)
  line L21 (95, 0) -> (99.7316, 13)
  line L22 (99.7316, 13) -> (102.2684, 13)
  line L23 (102.2684, 13) -> (107, 0)
  line L24 (107, 0) -> (112, 0)
  line L25 (112, 0) -> (116.7316, 13)
  line L26 (116.7316, 13) -> (119.2684, 13)
  line L27 (119.2684, 13) -> (124, 0)
  line L28 (124, 0) -> (129, 0)
  line L29 (129, 0) -> (133.7316, 13)
  line L30 (133.7316, 13) -> (136.2684, 13)
  line L31 (136.2684, 13) -> (141, 0)
  line L32 (141, 0) -> (146, 0)
  line L33 (146, 0) -> (150.7316, 13)
  line L34 (150.7316, 13) -> (153.2684, 13)
  line L35 (153.2684, 13) -> (158, 0)
  line L36 (158, 0) -> (163, 0)
  line L37 (163, 0) -> (167.7316, 13)
  line L38 (167.7316, 13) -> (170.2684, 13)
  line L39 (170.2684, 13) -> (175, 0)
  line L40 (175, 0) -> (180, 0)
  line L41 (180, 0) -> (184.7316, 13)
  line L42 (184.7316, 13) -> (187.2684, 13)
  line L43 (187.2684, 13) -> (192, 0)
  line L44 (192, 0) -> (197, 0)
  line L45 (197, 0) -> (201.7316, 13)
  line L46 (201.7316, 13) -> (204.2684, 13)
  line L47 (204.2684, 13) -> (209, 0)
  line L48 (209, 0) -> (214, 0)
  line L49 (214, 0) -> (218.7316, 13)
  line L50 (218.7316, 13) -> (221.2684, 13)
  line L51 (221.2684, 13) -> (226, 0)
  line L52 (226, 0) -> (231, 0)
  line L53 (231, 0) -> (235.7316, 13)
  line L54 (235.7316, 13) -> (238.2684, 13)
  line L55 (238.2684, 13) -> (243, 0)
  line L56 (243, 0) -> (250, 0)
  line L57 (250, 0) -> (250, 15)
  line L58 (250, 15) -> (0, 15)
  line L59 (0, 15) -> (0, 0)
  line L60 (22.6725, 4) -> (26.3275, 4)
  line L61 (26.3275, 4) -> (30.3312, 15)
  line L62 (22.6725, 4) -> (18.6688, 15)
  line L63 (18.6688, 15) -> (30.3312, 15)
  line L64 (39.6725, 4) -> (35.6688, 15)
  line L65 (39.6725, 4) -> (43.3275, 4)
  line L66 (43.3275, 4) -> (47.3312, 15)
  line L67 (35.6688, 15) -> (47.3312, 15)
  line L68 (56.6725, 4) -> (52.6688, 15)
  line L69 (56.6725, 4) -> (60.3275, 4)
  line L70 (60.3275, 4) -> (64.3312, 15)
  line L71 (52.6688, 15) -> (64.3312, 15)
  line L72 (73.6725, 4) -> (69.6688, 15)
  line L73 (73.6725, 4) -> (77.3275, 4)
  line L74 (77.3275, 4) -> (81.3312, 15)
  line L75 (69.6688, 15) -> (81.3312, 15)
  line L76 (90.6725, 4) -> (86.6688, 15)
  line L77 (90.6725, 4) -> (94.3275, 4)
  line L78 (94.3275, 4) -> (98.3312, 15)
  line L79 (86.6688, 15) -> (98.3312, 15)
  line L80 (107.6725, 4) -> (103.6688, 15)
  line L81 (107.6725, 4) -> (111.3275, 4)
  line L82 (111.3275, 4) -> (115.3312, 15)
  line L83 (103.6688, 15) -> (115.3312, 15)
  line L84 (124.6725, 4) -> (120.6688, 15)
  line L85 (124.6725, 4) -> (128.3275, 4)
  line L86 (128.3275, 4) -> (132.3312, 15)
  line L87 (120.6688, 15) -> (132.3312, 15)
  line L88 (141.6725, 4) -> (137.6688, 15)
  line L89 (141.6725, 4) -> (145.3275, 4)
  line L90 (145.3275, 4) -> (149.3312, 15)
  line L91 (137.6688, 15) -> (149.3312, 15)
  line L92 (158.6725, 4) -> (154.6688, 15)
  line L93 (158.6725, 4) -> (162.3275, 4)
  line L94 (162.3275, 4) -> (166.3312, 15)
  line L95 (154.6688, 15) -> (166.3312, 15)
  line L96 (175.6725, 4) -> (171.6688, 15)
  line L97 (175.6725, 4) -> (179.3275, 4)
  line L98 (179.3275, 4) -> (183.3312, 15)
  line L99 (171.6688, 15) -> (183.3312, 15)
  line L100 (192.6725, 4) -> (188.6688, 15)
  line L101 (192.6725, 4) -> (196.3275, 4)
  line L102 (196.3275, 4) -> (200.3312, 15)
  line L103 (188.6688, 15) -> (200.3312, 15)
  line L104 (209.6725, 4) -> (205.6688, 15)
  line L105 (209.6725, 4) -> (213.3275, 4)
  line L106 (213.3275, 4) -> (217.3312, 15)
  line L107 (205.6688, 15) -> (217.3312, 15)
  line L108 (226.6725, 4) -> (222.6688, 15)
  line L109 (226.6725, 4) -> (230.3275, 4)
  line L110 (230.3275, 4) -> (234.3312, 15)
  line L111 (222.6688, 15) -> (234.3312, 15)
  line L112 (4, 15) -> (4, 4)
  line L113 (4, 4) -> (9.3275, 4)
  line L114 (9.3275, 4) -> (13.3312, 15)
  line L115 (4, 15) -> (13.3312, 15)
  line L116 (247, 15) -> (247, 4)
  line L117 (247, 4) -> (243.6725, 4)
  line L118 (243.6725, 4) -> (239.6688, 15)
  line L119 (239.6688, 15) -> (247, 15)
  point P0 (34.2684, 13)
  point P1 (48.7316, 13)
  point P2 (51.2684, 13)
  point P3 (65.7316, 13)
  point P4 (68.2684, 13)
  point P5 (82.7316, 13)
  point P6 (85.2684, 13)
  point P7 (99.7316, 13)
  point P8 (102.2684, 13)
  point P9 (116.7316, 13)
  point P10 (119.2684, 13)
  point P11 (133.7316, 13)
  point P12 (136.2684, 13)
  point P13 (150.7316, 13)
  point P14 (153.2684, 13)
  point P15 (167.7316, 13)
  point P16 (170.2684, 13)
  point P17 (184.7316, 13)
  point P18 (187.2684, 13)
  point P19 (201.7316, 13)
  point P20 (204.2684, 13)
  point P21 (218.7316, 13)
  point P22 (221.2684, 13)
  point P23 (235.7316, 13)
  dimension "d94" = 4
  dimension "d95" = 2
  dimension "d96" = 2
  dimension "d99" = 17
  dimension "d100" = 0
  dimension "d101" = 4
  dimension "d102" = 4
  dimension "d103" = 2
  dimension "d104" = 3
  dimension "d105" = 4
  dimension "d106" = 2
  constraint coincident L58 L61.end
  constraint coincident L58 L62.end
  constraint parallel L3 L62
  constraint parallel L5 L61
  constraint parallel L4 L60
  constraint coincident L58 L112.start
  constraint perpendicular L58 L112
  constraint perpendicular L112 L113
  constraint coincident L58 L114.end
  constraint parallel L1 L114
  constraint coincident L58 L116.start
  constraint perpendicular L58 L116
  constraint perpendicular L116 L117
  constraint coincident L58 L118.end
  constraint parallel L55 L118
  measures "d94" distance of L4 L60
  measures "d95" distance of L3 L62
  measures "d96" distance of L5 L61
  measures "d101" distance of L59 L112
  measures "d102" distance of L0 L113
  measures "d103" distance of L1 L114
  measures "d104" distance of L57 L116
  measures "d105" distance of L56 L117
  measures "d106" distance of L55 L118
extrude "Extrude13" cut sketch "Sketch12" against normal blind 10 from surface at -3 contours L58 L112 L113 L114 L115 | L58 L60 L61 L62 L63 | L58 L64 L65 L66 L67 | L58 L68 L69 L70 L71 | L58 L72 L73 L74 L75 | L58 L76 L77 L78 L79 | L58 L80 L81 L82 L83 | L58 L84 L85 L86 L87 | L58 L88 L89 L90 L91 | L58 L92 L93 L94 L95 | L58 L96 L97 L98 L99 | L58 L100 L101 L102 L103 | L58 L104 L105 L106 L107 | L58 L108 L109 L110 L111 | L58 L116 L117 L118 L119 bodies 39
ref_plane "WorkPlane3" through (275, 125, 7.5) normal (1, 0, 0) x (0, 0, -1)
mirror "Mirror2" about plane through (275, 125, 7.5) normal (1, 0, 0) of "Extrude13"